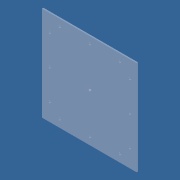
# Autodesk Inventor part: J007125
Saved by Autodesk Inventor 2018.2 (Build 222227000, 227)
## iProperties
Created: 2014-04-25
Material: ACRYLIC, WHITE 2447
Vendor: HHMI: JFRC - ID&F
Document SubType Name: Modeling
Designer: NEGRASHOVI
Density: 0.66 g/cm^3
Mass: 369.82 g
Surface Area: 961.375 cm^2
Volume: 147.339 cm^3
Part Number: J007125
Description: CHAMBER BOTTOM GLASS
Appearance: Polycarbonate (Clear)
Project: P-298001
RuleStatus: InUse
AfterDocSave0: file://Part Number Cleaner
LAB/DEPT: RUBIN (LAB)
REQUESTING SCIENTIST: ASO, YOSHI
SURFACE ROUGHNESS: N/A
DESIGN DEPARTMENT: HHMI: JRC - ID&F
SPECIAL FINISH: NONE
ALTERED ITEM PART NUMBER: N/A
ALTERED ITEM VENDOR: N/A
ALTERED ITEM DESCRIPTION: N/A
Revision Number: B
Autodesk Inventor part; units mm, degrees
ref_plane "YZ Plane" through (0, 0, 0) normal (1, 0, 0) x (0, 1, 0)
ref_plane "XZ Plane" through (0, 0, 0) normal (0, 1, 0) x (-1, 0, 0)
ref_plane "XY Plane" through (0, 0, 0) normal (0, 0, 1) x (1, 0, 0)
sketch "Sketch1" plane through (0, 0, 0) normal (0, 0, 1) x (1, 0, 0)
  line L0 (-107.95, -107.95) -> (107.95, -107.95)
  line L1 (107.95, -107.95) -> (107.95, 107.95)
  line L2 (107.95, 107.95) -> (-107.95, 107.95)
  line L3 (-107.95, 107.95) -> (-107.95, -107.95)
  line L4 (-107.95, -107.95) -> (107.95, 107.95) construction
  point P0 (0, 0)
  point P1 (0, 0)
  dimension "d0" = 215.9
  dimension "d1" = 215.9
  constraints: 10 end point, 2 parallel, 1 coincident, 1 horizontal, 1 midpoint, 1 perpendicular
  measures "d0" distance of L1.end L2.end
  measures "d1" distance of L2.end L0.start
extrude "Extrusion1" add sketch "Sketch1" along normal blind 3.175
sketch "Sketch2" plane through (0, 0, 3.175) normal (0, 0, 1) x (1, 0, 0)
  line L0 (-91.44, -91.44) -> (91.44, -91.44) construction
  line L1 (91.44, -91.44) -> (91.44, 91.44) construction
  line L2 (91.44, 91.44) -> (-91.44, 91.44) construction
  line L3 (-91.44, 91.44) -> (-91.44, -91.44) construction
  line L4 (-91.44, -91.44) -> (91.44, 91.44) construction
  line L5 (-151.13, 0) -> (151.13, 0) construction
  line L6 (0, -151.13) -> (0, 151.13) construction
  point P0 (0, 0)
  point P1 (0, 0)
  point P2 (-68.58, 91.44)
  point P3 (0, 91.44)
  point P4 (68.58, 91.44)
  point P5 (91.44, 68.58)
  point P6 (91.44, 0)
  point P7 (68.58, -91.44)
  point P8 (0, -91.44)
  point P9 (-68.58, -91.44)
  point P10 (-91.44, -68.58)
  point P11 (-91.44, 0)
  point P12 (-91.44, 68.58)
  point P13 (91.44, -68.58)
  dimension "d4" = 182.88
  dimension "d5" = 182.88
  dimension "d6" = 22.86
  dimension "d7" = 22.86
  constraints: 12 point on line, 10 end point, 6 symmetric about line, 5 midpoint, 2 parallel, 1 coincident, 1 horizontal, 1 perpendicular
  measures "d4" distance of L1.end L2.end
  measures "d5" distance of L0.end L1.end
  measures "d6" distance from line of point (-68.58, 91.44) L3
  measures "d7" distance from line of point (-91.44, 68.58) L2
hole "Hole1" at (-68.58, 91.44, 3.175) at (0, 91.44, 3.175) at (68.58, 91.44, 3.175) at (91.44, 68.58, 3.175) at (91.44, 0, 3.175) at (68.58, -91.44, 3.175) at (0, -91.44, 3.175) at (-68.58, -91.44, 3.175) at (-91.44, -68.58, 3.175) at (-91.44, 0, 3.175) at (-91.44, 68.58, 3.175) at (91.44, -68.58, 3.175) direction (0, 0, -1) diameter 4.7625 end through all clearance for "Flat Head Machine Screw (82)" size "#8" standard "Ansi Unified Screw Threads"
sketch "Sketch3" plane through (0, 0, 3.175) normal (0, 0, 1) x (1, 0, 0)
  line L0 (-1.27, -0.7332) -> (-1.27, 0.7332) construction
  line L1 (-1.27, 0.7332) -> (0, 1.4665) construction
  line L2 (0, 1.4665) -> (1.27, 0.7332) construction
  line L3 (1.27, 0.7332) -> (1.27, -0.7332) construction
  line L4 (1.27, -0.7332) -> (0, -1.4665) construction
  line L5 (0, -1.4665) -> (-1.27, -0.7332) construction
  point P0 (0, 0)
  point P1 (0, 0)
  point P2 (0, 0)
  dimension "d23" = 2.54
  constraints: 12 end point, 8 coincident, 1 vertical, 13 other
  measures "d23" distance between parallel lines of L0 L3
hole "Hole2" at (0, 0, 3.175) at (0, 1.4665, 3.175) at (1.27, 0.7332, 3.175) at (1.27, -0.7332, 3.175) at (0, -1.4665, 3.175) at (-1.27, -0.7332, 3.175) at (-1.27, 0.7332, 3.175) direction (0, 0, -1) diameter 0.8 end through all
body "Solid1"
